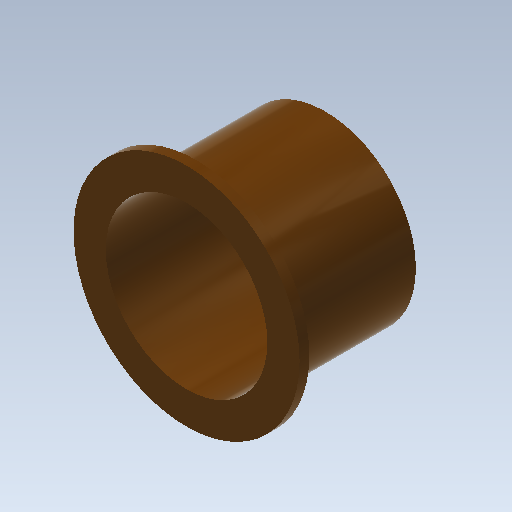
# Autodesk Inventor part: H4FM_2528_21
Saved by Autodesk Inventor 2020 (Build 240168000, 168)
## iProperties
Created: 2016-11-11
Part Number: H4FM_2528_21
Material: Generic
Document SubType Name: Modeling
Designer: jous
Density: 1 g/cm^3
Appearance: Default
Mass: 3.20442 g
Surface Area: 45.5531 cm^2
Volume: 3.20442 cm^3
Author: jous
Autodesk Inventor part; units mm, degrees
ref_plane "YZ Plane" through (0, 0, 0) normal (1, 0, 0) x (0, 1, 0)
ref_plane "XZ Plane" through (0, 0, 0) normal (0, 1, 0) x (-1, 0, 0)
ref_plane "XY Plane" through (0, 0, 0) normal (0, 0, 1) x (1, 0, 0)
sketch "Sketch1" plane through (0, 0, 0) normal (0, 0, 1) x (1, 0, 0)
  circle A0 centre (0, 0) radius 12.5
  circle A1 centre (0, 0) radius 14
  dimension "d0" = 25
  dimension "d1" = 28
  constraints: 2 centre point, 2 coincident
  measures "d0" diameter of A0
  measures "d1" diameter of A1
extrude "Extrusion1" add sketch "Sketch1" along normal blind 20
sketch "Sketch2" plane through (0, 0, 20) normal (0, 0, 1) x (1, 0, 0)
  circle A0 centre (0, 0) radius 12.5 projected
  circle A1 centre (0, 0) radius 14 projected
  circle A2 centre (0, 0) radius 12.5
  circle A3 centre (0, 0) radius 17.5
  dimension "d4" = 35
  constraints: 2 centre point, 2 coincident, 1 concentric
  measures "d4" diameter of A3
extrude "Extrusion2" add sketch "Sketch2" along normal blind 1.5 contours A1 | A3
body "Solid1"
